surface mount (Autodesk Fusion 360 design; units mm, degrees)
Autodesk Fusion 360 part; units mm, degrees
sketch "Sketch1" plane through (0, 0, 0) normal (0, 1, 0) x (1, 0, 0)
  line L0 (0, 0) -> (290, 0)
  line L1 (290, 0) -> (290, -90)
  line L2 (290, -90) -> (0, -90)
  line L3 (0, -90) -> (0, 0)
  line L4 (-2, 2) -> (292, 2)
  line L5 (292, 2) -> (292, -92)
  line L6 (292, -92) -> (-2, -92)
  line L7 (-2, -92) -> (-2, 2)
  line L8 (0, 0) -> (292, 0)
  line L9 (292, 0) -> (292, -92)
  line L10 (292, -92) -> (0, -92)
  line L11 (0, -92) -> (0, 0)
  line L12 (290, -90) -> (0, -90)
  line L13 (0, -90) -> (0, 0)
  line L14 (0, 0) -> (290, 0)
  line L15 (290, 0) -> (290, -90)
  line L16 (290, -90) -> (0, -90)
  line L17 (0, -90) -> (0, -92)
  line L18 (0, -92) -> (290, -92)
  line L19 (290, -92) -> (290, -90)
  line L20 (287, -87) -> (3, -87)
  line L21 (3, -87) -> (3, -3)
  line L22 (3, -3) -> (287, -3)
  line L23 (287, -3) -> (287, -87)
  dimension "d1" = 290
  dimension "d2" = 90
  dimension "d3" = 2
  dimension "d4" = 3
  constraint horizontal L0
  constraint vertical L1
  constraint horizontal L2
  constraint vertical L3
  constraint coincident L0.start L3.end
  constraint horizontal L8
  constraint vertical L9
  constraint horizontal L10
  constraint vertical L11
  constraint horizontal L12
  constraint vertical L13
  constraint horizontal L14
  constraint vertical L15
  constraint horizontal L16
  constraint vertical L17
  constraint horizontal L18
  constraint vertical L19
  measures "d1" distance of L0.start L0.end
  measures "d2" distance of L0.start L2.end
extrude "Extrude1" add sketch "Sketch1" along normal blind 5 contours L0 L3 L4 L5 L6 L7 L8 L11 L13 L14 L17 makes body 1
extrude "Extrude2" add sketch "Sketch1" along normal blind 2.5 contours L0 L1 L2 L3 L8 L11 L12 L13 L14 L15 L16 bodies 1
sketch "Sketch2" plane through (0, 0, 0) normal (0, 1, 0) x (1, 0, 0)
  circle A0 centre (3, -87) radius 15
  circle A1 centre (287, -87) radius 15
  line L0 (3, -87) -> (3, -72)
  line L1 (3, -87) -> (18, -87)
  line L2 (287, -87) -> (272, -87)
  line L3 (287, -87) -> (287, -72)
  point P0 (3, -87)
  point P1 (287, -87)
  dimension "d9" = 30
  dimension "d10" = 30
  constraint coincident P0 A0.centre
  constraint coincident P1 A1.centre
  constraint coincident A0 L0.end
  constraint coincident A0 L1.end
  constraint perpendicular L0 L1
  constraint coincident A1 L2.end
  constraint parallel L1 L2
  constraint coincident A1 L3.end
  constraint perpendicular L2 L3
  measures "d9" diameter of A0
  measures "d10" diameter of A1
extrude "Extrude4" add sketch "Sketch2" along normal blind 2.5 contours A0 L0 L1 | A1 L2 L3 picked at (12.3456, -83.5143) picked at (283.5143, -77.6544) bodies 1
extrude "Extrude3" add sketch "Sketch1" along normal blind 5 contours L1 L5 L6 L8 L9 L10 L15 L19 bodies 1
sketch "Sketch3" plane through (0, 0, 0) normal (0, 1, 0) x (1, 0, 0)
  line L0 (-2, 2) -> (292, 2)
  line L1 (292, -92) -> (292, 2)
  line L2 (-2, -92) -> (-2, 2)
  line L3 (292, -45) -> (-2, -45)
  line L4 (292, -92) -> (-2, -92)
  line L5 (145, -45) -> (145, -92)
  line L6 (145, -45) -> (145, 2)
  point P0 (292, -92)
  point P1 (292, 2)
  constraint coincident P0 L1.start
  constraint coincident P1 L0.end
  constraint midpoint L1 L3.start
  constraint midpoint L2 L3.end
  constraint midpoint L3 L5.start
  constraint midpoint L4 L5.end
  constraint midpoint L0 L6.end
extrude "Extrude5" cut sketch "Sketch3" along normal blind 10 contours L0 L1 L3 L6 | L1 L3 L4 L5 bodies 1
sketch "Sketch4" plane through (0, 0, 0) normal (0, -1, 0) x (1, 0, 0)
  line L0 (145, -2) -> (145, 3)
  line L1 (145, 3) -> (3, 3)
  line L2 (3, 3) -> (3, 72)
  arc A0 (3, 72) -> (18, 87) centre (3, 87) ccw
  line L3 (18, 87) -> (145, 87)
  line L4 (145, 87) -> (145, 90)
  line L5 (145, 90) -> (0, 90)
  line L6 (0, 90) -> (0, 92)
  line L7 (0, 92) -> (-2, 92)
  line L8 (-2, 92) -> (-2, -2)
  line L9 (-2, -2) -> (145, -2)
  circle A1 centre (3, 3) radius 15
  line L10 (3, 18) -> (3, 3)
  line L11 (18, 3) -> (3, 3)
  dimension "d17" = 30
  constraint coincident L1.end L2.start
  constraint coincident A1 L10.start
  constraint coincident L2 L10.start
  constraint coincident A1 L11.start
  constraint coincident L1 L11.start
  measures "d17" diameter of A1
extrude "Extrude6" add sketch "Sketch4" against normal blind 2.5 contours L1 L2 A1 L10 L11 bodies 1
move_face "OffsetFaces1" offset -127 1 faces at (145, 0.8333, 0.3333) on bodies 1
move_face "OffsetFaces2" offset -127 1 faces at (145, 0.8333, 88) on bodies 1
sketch "Sketch5" plane through (-2, 0, 0) normal (-1, 0, 0) x (0, 0, 1)
  line L0 (-2, 0) -> (92, 0)
  line L1 (92, 0) -> (92, 5)
  line L2 (92, 5) -> (-2, 5)
  line L3 (-2, 5) -> (-2, 0)
  line L4 (-2, 5) -> (92, 5)
  line L5 (92, 5) -> (92, 0)
  line L6 (92, 0) -> (-2, 0)
  line L7 (-2, 0) -> (-2, 5)
  constraint horizontal L4
  constraint vertical L5
  constraint horizontal L6
  constraint vertical L7
  constraint coincident L0.end L1.start
  constraint coincident L2.end L3.start
extrude "Extrude7" add sketch "Sketch5" along normal blind 10 bodies 1
extrude "Extrude8" add 1 faces at (-7, 0, 54) along direction (0, -1, 0) blind 2.5 on bodies 1 bodies 1
fillet "Fillet1" radius 10 1 edges at (0, 1.25, 92) on bodies 1
sketch "Sketch6" plane through (0, -2.5, 0) normal (0, -1, 0) x (1, 0, 0)
  line L0 (18, 90) -> (-4, 90)
  arc A0 (-4, 90) -> (-10, 92) centre (-10, 82) ccw
  line L1 (-10, 92) -> (-12, 92)
  line L2 (-12, 92) -> (-12, -2)
  line L3 (-12, -2) -> (18, -2)
  line L4 (18, -2) -> (18, 3)
  arc A1 (18, 3) -> (3, 18) centre (3, 3) ccw
  line L5 (3, 18) -> (3, 72)
  arc A2 (3, 72) -> (18, 87) centre (3, 87) ccw
  line L6 (18, 87) -> (18, 90)
  line L7 (18, 90) -> (18, -2)
  constraint coincident L0.start L6.end
  constraint coincident L3.end L4.start
extrude "Extrude9" add sketch "Sketch6" against normal blind 5 contours A1 L5 A2 L7 bodies 1
extrude "Extrude10" add 1 faces at (8, 0, -2) along direction (0, 0, -1) blind 3 on bodies 1 bodies 1
sketch "Sketch7" plane through (-12, 0, 0) normal (-1, 0, 0) x (0, 0, 1)
  line L0 (92, -2.5) -> (92, 5)
  line L1 (92, 5) -> (-5, 5)
  line L2 (-5, 5) -> (-5, -2.5)
  line L3 (-5, -2.5) -> (92, -2.5)
sketch "Sketch8" plane through (0, 5, 0) normal (0, 1, 0) x (-1, 0, 0)
  arc A0 (10, 92) -> (0, 82) centre (10, 82) ccw
  line L0 (0, 82) -> (0, 0)
  line L1 (0, 0) -> (-18, 0)
  line L2 (-18, 0) -> (-18, -5)
  line L3 (-18, -5) -> (12, -5)
  line L4 (12, -5) -> (12, 92)
  line L5 (12, 92) -> (10, 92)
  line L6 (12, -5) -> (6, -5)
  circle A1 centre (6, 15) radius 1.5
  circle A2 centre (6, 35) radius 1.5
  circle A3 centre (6, 55) radius 1.5
  circle A4 centre (6, 75) radius 1.5
  dimension "d31" = 6
  dimension "d33" = 20
  dimension "d34" = 20
  dimension "d35" = 20
  dimension "d36" = 20
  dimension "d37" = 3
  dimension "d38" = 3
  dimension "d39" = 3
  dimension "d40" = 3
  constraint coincident L3.end L4.start
  measures "d31" distance of L3.end L6.end
  measures "d33" distance of L6.end A1.centre
  measures "d34" distance of A1.centre A2.centre
  measures "d35" distance of A2.centre A3.centre
  measures "d36" distance of A3.centre A4.centre
  measures "d37" diameter of A1
  measures "d38" diameter of A2
  measures "d39" diameter of A3
  measures "d40" diameter of A4
extrude "Extrude11" cut sketch "Sketch8" against normal blind 15 contours A1 | A2 | A3 | A4 bodies 1
sketch "Sketch9" plane through (0, -2.5, 0) normal (0, -1, 0) x (1, 0, 0)
  circle A0 centre (-6, 35) radius 1.5
  circle A1 centre (-6, 55) radius 1.5
  circle A2 centre (-6, 15) radius 1.5
  circle A3 centre (-6, 75) radius 1.5
  line L0 (18, 90) -> (-4, 90)
  arc A4 (-4, 90) -> (-10, 92) centre (-10, 82) ccw
  line L1 (-10, 92) -> (-12, 92)
  line L2 (-12, 92) -> (-12, -5)
  line L3 (-12, -5) -> (18, -5)
  line L4 (18, -5) -> (18, 90)
  circle A5 centre (-6, 75) radius 3
  circle A6 centre (-6, 55) radius 1.5
  circle A7 centre (-6, 55) radius 3
  circle A8 centre (-6, 35) radius 3
  circle A9 centre (-6, 15) radius 3
  dimension "d49" = 6
  dimension "d50" = 3
  dimension "d51" = 6
  dimension "d52" = 6
  dimension "d53" = 6
  constraint concentric A3 A5
  constraint concentric A1 A6
  constraint concentric A1 A7
  constraint concentric A0 A8
  constraint concentric A2 A9
  measures "d49" diameter of A5
  measures "d50" diameter of A6
  measures "d51" diameter of A7
  measures "d52" diameter of A8
  measures "d53" diameter of A9
extrude "Extrude13" cut sketch "Sketch9" against normal blind 2 contours A5 | A7 | A8 | A9 bodies 1
fillet "Fillet2" radius 50 1 edges at (18, 0, 90) on bodies 1
fillet "Fillet3" radius 5 1 edges at (-12, 1.25, -5) on bodies 1
fillet "Fillet4" radius 3 1 edges at (18, 1.25, -5) on bodies 1
fillet "Fillet5" radius 1 4 edges at (-4.6015, -0.5, 15.5424) (-4.6015, -0.5, 35.5424) (-4.6015, -0.5, 55.5424) (-4.6015, -0.5, 75.5424) on bodies 1
fillet "Fillet6" radius 1 4 edges at (-8.797, -2.5, 16.0848) (-8.797, -2.5, 36.0848) (-8.797, -2.5, 56.0848) (-8.797, -2.5, 76.0848) on bodies 1
fillet "Fillet7" radius 4 1 edges at (-12, 1.25, 92) on bodies 1
fillet "Fillet8" radius 3 2 edges at (18, 2.5, 24.2877) (12.1588, 2.5, 72.0274) on bodies 1
copy_body "Body->Comp1" bodies 1 removing the originals makes body 2 in component "Component"
mirror "Mirror1" about plane through (0, 0, 0) normal (1, 0, 0) of bodies 2 makes body 3 in component "Component"
move_body "Move1" bodies 3 to x (1, 0, 0) y (0, 1, 0) z (0, 0, 1) at (38, 0, 0) in component "Component"
component "Component" placed x (1, 0, 0) y (0, 1, 0) z (0, 0, 1) at (0, 0, 0)
